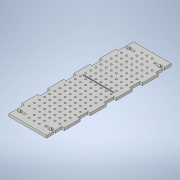
# Autodesk Inventor part: V3 Mounting Plate
Saved by Autodesk Inventor 2022.1 (Build 261234020, 234B)
## iProperties
Created: 2020-05-07
Part Number: V3 Mounting Plate
Material: Generic
Document SubType Name: Modeling
Designer: Workshop Tech
Density: 1 g/cm^3
Appearance: Default
Author: Workshop Tech
Autodesk Inventor part; units mm, degrees
ref_plane "YZ Plane" through (0, 0, 0) normal (1, 0, 0) x (0, 1, 0)
ref_plane "XZ Plane" through (0, 0, 0) normal (0, 1, 0) x (-1, 0, 0)
ref_plane "XY Plane" through (0, 0, 0) normal (0, 0, 1) x (1, 0, 0)
sketch "Sketch1" plane through (0, 0, 0) normal (0, 1, 0) x (-1, 0, 0)
  line L0 (0, 0) -> (104.96, 0)
  line L1 (104.96, 0) -> (104.96, -308.6568)
  line L2 (104.96, -308.6568) -> (0, -308.6568)
  line L3 (0, -308.6568) -> (0, 0)
  dimension "d0" = 104.96
  dimension "d1" = 308.6568
  constraints: 8 end point, 2 parallel, 1 horizontal, 1 perpendicular
  measures "d0" distance between parallel lines of L3 L1
  measures "d1" distance between parallel lines of L2 L0
extrude "Base" add sketch "Sketch1" along normal blind 6
sketch "Sketch7" plane through (0, 6, 0) normal (0, 1, 0) x (1, 0, 0)
  line L0 (0, 0) -> (0, 308.6568) projected
  line L1 (-104.96, 0) -> (0, 0) projected
  line L2 (-104.96, 0) -> (0, 0) projected
  line L3 (0, 0) -> (0, 308.6568) projected
  line L4 (0, 308.6568) -> (-104.96, 308.6568) projected
  line L5 (-104.96, 308.6568) -> (-104.96, 0) projected
  point P0 (-52.48, 270.5568)
  dimension "d35" = 38.1
  dimension "d36" = 52.48
  measures "d35" distance from line of L4 point (-52.48, 270.557)
  measures "d36" distance from line of L5 point (-52.48, 270.557)
hole "Board Hole" at (-52.48, 6, -270.5568) direction (0, -1, 0) diameter 4.25 end through all clearance for "Flat Head Machine Screw" size "M4" standard "Ansi Metric M Profile"
pattern_linear "Patterned Board Holes" count 19 spacing 12.7 along (0, 0, 1) count 7 spacing 12.7 along (1, 0, 0) of "Board Hole" second direction both ways yes
sketch "Sketch12" plane through (0, 6, 0) normal (0, 1, 0) x (1, 0, 0)
  line L0 (0, 308.6568) -> (0, 0) projected
  line L1 (-104.96, 0) -> (-104.96, 308.6568) projected
  line L2 (0, 0) -> (-5.875, 0)
  line L3 (-5.875, 0) -> (-5.875, 38.04)
  line L4 (-5.875, 38.04) -> (0, 38.04)
  line L5 (0, 38.04) -> (0, 0)
  line L6 (-104.96, 0) -> (0, 0) projected
  line L7 (-104.96, 0) -> (-99.085, 0)
  line L8 (-99.085, 0) -> (-99.085, 38.04)
  line L9 (-99.085, 38.04) -> (-104.96, 38.04)
  line L10 (-104.96, 38.04) -> (-104.96, 0)
  point P0 (0, 38.04)
  dimension "d188" = 5.875
  dimension "d189" = 38.04
  dimension "d190" = 5.875
  dimension "d191" = 38.04
  constraints: 16 end point, 4 parallel, 2 horizontal, 2 perpendicular
  measures "d188" distance of L3.end L4.end
  measures "d189" distance of L2.end L3.end
  measures "d190" distance of L9.end L8.end
  measures "d191" distance of L8.end L7.end
extrude "Extrusion4" cut sketch "Sketch12" against normal blind 25.4
sketch "Sketch13" plane through (0, 6, 0) normal (0, 1, 0) x (1, 0, 0)
  line L0 (0, 0) -> (0, 308.6568) projected
  line L1 (0, 308.6568) -> (-5.875, 308.6568)
  line L2 (-5.875, 270.6168) -> (0, 270.6168)
  line L3 (-5.875, 270.6168) -> (-5.875, 308.6568)
  line L4 (0, 308.6568) -> (0, 0) projected
  line L5 (0, 270.6168) -> (0, 308.6568)
  line L6 (0, 308.6568) -> (-104.96, 308.6568) projected
  line L7 (-104.96, 308.6568) -> (-99.085, 308.6568)
  line L8 (-99.085, 308.6568) -> (-99.085, 270.6168)
  line L9 (-99.085, 270.6168) -> (-104.96, 270.6168)
  line L10 (-104.96, 270.6168) -> (-104.96, 308.6568)
  point P0 (0, 38.1)
  point P1 (0, 270.6168)
  dimension "d175" = 38.04
  dimension "d176" = 5.875
  dimension "d178" = 5.875
  dimension "d179" = 38.04
  constraints: 16 end point, 2 horizontal, 2 parallel, 1 collinear, 1 perpendicular, 1 vertical
  measures "d175" distance of L2.start L1.end
  measures "d176" distance of L2.start L2.end
  measures "d178" distance of L8.end L9.end
  measures "d179" distance of L7.end L8.end
sketch "Sketch16" plane through (0, 6, 0) normal (0, 1, 0) x (1, 0, 0)
  circle A0 centre (-52.48, 270.5568) radius 2.125 projected
  point P0 (0, 0)
  point P1 (-52.48, 283.2568)
  dimension "d163" = 12.7
  measures "d163" distance of A0.centre point (-52.48, 283.257)
hole "Hole9" at (-52.48, 6, -283.2568) direction (0, -1, 0) diameter 4.25 end through all clearance for "Flat Head Machine Screw" size "M4" standard "Ansi Metric M Profile"
sketch "Sketch17" plane through (0, 6, 0) normal (0, 1, 0) x (1, 0, 0)
  line L0 (0, 38.04) -> (0, 308.6568) projected
  line L1 (-99.085, 0) -> (-5.875, 0) projected
  line L2 (0, 308.6568) -> (-104.96, 308.6568) projected
  line L3 (-5.875, 141.8134) -> (0, 141.8134)
  line L4 (0, 141.8134) -> (0, 166.8434)
  line L5 (0, 166.8434) -> (-5.875, 166.8434)
  line L6 (-5.875, 166.8434) -> (-5.875, 141.8134)
  line L7 (-52.48, 0) -> (-52.48, 308.6568)
  line L8 (-5.875, 206.2151) -> (0, 206.2151)
  line L9 (0, 206.2151) -> (0, 231.2451)
  line L10 (0, 231.2451) -> (-5.875, 231.2451)
  line L11 (-5.875, 231.2451) -> (-5.875, 206.2151)
  line L12 (-5.875, 77.4117) -> (0, 77.4117)
  line L13 (0, 77.4117) -> (0, 102.4417)
  line L14 (0, 102.4417) -> (-5.875, 102.4417)
  line L15 (-5.875, 102.4417) -> (-5.875, 77.4117)
  line L16 (-99.085, 141.8134) -> (-104.96, 141.8134)
  line L17 (-104.96, 141.8134) -> (-104.96, 166.8434)
  line L18 (-104.96, 166.8434) -> (-99.085, 166.8434)
  line L19 (-99.085, 166.8434) -> (-99.085, 141.8134)
  line L20 (-104.96, 231.2451) -> (-99.085, 231.2451)
  line L21 (-99.085, 231.2451) -> (-99.085, 206.2151)
  line L22 (-104.96, 206.2151) -> (-104.96, 231.2451)
  line L23 (-99.085, 206.2151) -> (-104.96, 206.2151)
  line L24 (-104.96, 102.4417) -> (-99.085, 102.4417)
  line L25 (-99.085, 102.4417) -> (-99.085, 77.4117)
  line L26 (-104.96, 77.4117) -> (-104.96, 102.4417)
  line L27 (-99.085, 77.4117) -> (-104.96, 77.4117)
  point P0 (-52.48, 154.3284)
  point P1 (-5.875, 154.3284)
  point P2 (-52.48, 154.3284)
  point P3 (0, 154.3284)
  point P4 (-5.875, 218.7301)
  point P5 (0, 218.7301)
  point P6 (-5.875, 89.9267)
  point P7 (0, 89.9267)
  point P8 (-104.96, 102.6267)
  point P9 (-104.96, 231.4301)
  point P10 (-99.085, 154.3284)
  point P11 (-104.96, 154.3284)
  point P12 (-99.085, 218.7301)
  point P13 (-104.96, 218.7301)
  point P14 (-99.085, 89.9267)
  point P15 (-104.96, 89.9267)
  dimension "d257" = 5.875
  dimension "d258" = 25.03
  dimension "d259" = 5.875
  dimension "d260" = 25.03
  dimension "d261" = 5.875
  dimension "d262" = 25.03
  dimension "d264" = 89.9267
  dimension "d266" = 89.9267
  dimension "d269" = 154.3284
  dimension "d270" = 52.48
  constraints: 50 end point, 18 symmetric about line, 9 midpoint, 6 parallel, 3 horizontal, 3 perpendicular, 3 point on line, 1 horizontal alignment
  measures "d257" distance of L5.end L4.end
  measures "d258" distance of L4.end L3.end
  measures "d259" distance of L10.end L10.start
  measures "d260" distance of L10.start L9.start
  measures "d261" distance of L14.end L14.start
  measures "d262" distance of L14.start L13.start
  measures "d264" distance from line of L2 point (0, 218.73)
  measures "d266" distance from line of L1 point (-5.875, 89.927)
  measures "d269" distance from line of point (-52.48, 154.328) L2
  measures "d270" distance from line of point (-52.48, 154.328) L0
extrude "Extrusion6" cut sketch "Sketch17" against normal blind 25.4
extrude "Extrusion7" cut sketch "Sketch13" against normal blind 25.4
sketch "Sketch18" plane through (0, 6, 0) normal (0, 1, 0) x (1, 0, 0)
  line L0 (0, 291.6047) -> (0, 287.1089) projected
  line L1 (0, 291.6047) -> (0, 287.1089) projected
  line L2 (-28.125, 287.2339) -> (-28.125, 291.7297)
  line L3 (0, 291.7297) -> (0, 287.1089)
  line L4 (-16.25, 285.2943) -> (-12, 285.2943)
  line L5 (-12, 293.5443) -> (-16.25, 293.5443)
  line L6 (0, 287.1089) -> (-12, 287.1089)
  line L7 (-16.25, 287.2339) -> (-28.125, 287.2339)
  line L8 (-28.125, 291.7297) -> (-16.25, 291.7297)
  line L9 (-12, 291.7297) -> (0, 291.7297)
  line L10 (-16.25, 293.5443) -> (-16.25, 291.7297)
  line L11 (-16.25, 287.2339) -> (-16.25, 285.2943)
  line L12 (-12, 285.2943) -> (-12, 287.1089)
  line L13 (-12, 291.7297) -> (-12, 293.5443)
  line L14 (-5.875, 308.6568) -> (-99.085, 308.6568) projected
  line L15 (-99.085, 38.04) -> (-99.085, 0) projected
  line L16 (-99.085, 308.6568) -> (-99.085, 270.6168) projected
  line L17 (-52.48, 308.6568) -> (-52.48, 0)
  line L18 (-142.1882, 0) -> (-142.1882, 308.6568)
  line L19 (-142.1882, 154.3284) -> (31.2958, 154.3284)
  line L20 (-104.96, 291.6047) -> (-104.96, 287.1089)
  line L21 (-104.96, 291.6047) -> (-104.96, 287.1089)
  line L22 (-76.835, 287.2339) -> (-76.835, 291.7297)
  line L23 (-104.96, 291.7297) -> (-104.96, 287.1089)
  line L24 (-88.71, 285.2943) -> (-92.96, 285.2943)
  line L25 (-92.96, 293.5443) -> (-88.71, 293.5443)
  line L26 (-104.96, 287.1089) -> (-92.96, 287.1089)
  line L27 (-88.71, 287.2339) -> (-76.835, 287.2339)
  line L28 (-76.835, 291.7297) -> (-88.71, 291.7297)
  line L29 (-92.96, 291.7297) -> (-104.96, 291.7297)
  line L30 (-88.71, 293.5443) -> (-88.71, 291.7297)
  line L31 (-88.71, 287.2339) -> (-88.71, 285.2943)
  line L32 (-92.96, 285.2943) -> (-92.96, 287.1089)
  line L33 (-92.96, 291.7297) -> (-92.96, 293.5443)
  line L34 (-99.085, 308.6568) -> (-5.875, 308.6568)
  line L35 (0, 17.0521) -> (0, 21.5479)
  line L36 (0, 17.0521) -> (0, 21.5479)
  line L37 (-28.125, 21.4229) -> (-28.125, 16.9271)
  line L38 (0, 16.9271) -> (0, 21.5479)
  line L39 (-16.25, 23.3625) -> (-12, 23.3625)
  line L40 (-12, 15.1125) -> (-16.25, 15.1125)
  line L41 (0, 21.5479) -> (-12, 21.5479)
  line L42 (-16.25, 21.4229) -> (-28.125, 21.4229)
  line L43 (-28.125, 16.9271) -> (-16.25, 16.9271)
  line L44 (-12, 16.9271) -> (0, 16.9271)
  line L45 (-16.25, 15.1125) -> (-16.25, 16.9271)
  line L46 (-16.25, 21.4229) -> (-16.25, 23.3625)
  line L47 (-12, 23.3625) -> (-12, 21.5479)
  line L48 (-12, 16.9271) -> (-12, 15.1125)
  line L49 (-99.085, 0) -> (-99.085, 38.04)
  line L50 (-76.835, 16.9271) -> (-88.71, 16.9271)
  line L51 (-76.835, 21.4229) -> (-76.835, 16.9271)
  line L52 (-88.71, 21.4229) -> (-76.835, 21.4229)
  line L53 (-92.96, 15.1125) -> (-88.71, 15.1125)
  line L54 (-92.96, 16.9271) -> (-92.96, 15.1125)
  line L55 (-88.71, 21.4229) -> (-88.71, 23.3625)
  line L56 (-92.96, 23.3625) -> (-92.96, 21.5479)
  line L57 (-88.71, 23.3625) -> (-92.96, 23.3625)
  line L58 (-92.96, 16.9271) -> (-104.96, 16.9271)
  line L59 (-104.96, 21.5479) -> (-92.96, 21.5479)
  line L60 (-104.96, 17.0521) -> (-104.96, 21.5479)
  line L61 (-104.96, 17.0521) -> (-104.96, 21.5479)
  line L62 (-104.96, 16.9271) -> (-104.96, 21.5479)
  line L63 (-88.71, 15.1125) -> (-88.71, 16.9271)
  point P0 (-5.875, 270.6168)
  point P1 (-19.9732, 289.3568)
  point P2 (0, 289.3568)
  point P3 (0, 289.3568)
  point P4 (-84.9868, 289.3568)
  point P5 (-104.96, 289.3568)
  point P6 (-104.96, 289.3568)
  point P7 (-5.875, 38.04)
  point P8 (-19.9732, 19.3)
  point P9 (0, 19.3)
  point P10 (0, 19.3)
  point P11 (-84.9868, 19.3)
  point P12 (-104.96, 19.3)
  point P13 (-104.96, 19.3)
  dimension "d237" = 28.125
  dimension "d238" = 4.25
  dimension "d239" = 8.25
  dimension "d240" = 12
  dimension "d242" = 16.9271
  dimension "d256" = 4.4958
  constraints: 118 end point, 52 symmetric about line, 10 parallel, 8 midpoint, 4 horizontal, 4 perpendicular, 2 equal length, 1 horizontal alignment, 1 vertical
  measures "d237" distance of L2.end L3.start
  measures "d238" distance of L5.end L5.start
  measures "d239" distance of L5.start L4.end
  measures "d240" distance of L9.start L3.start
  measures "d242" distance between parallel lines of L14 L9
  measures "d256" distance between parallel lines of L8 L7
extrude "Extrusion8" cut sketch "Sketch18" against normal blind 25.4
pattern_linear "Rectangular Pattern6" count 2 spacing 12.7 along (0, 0, -1) count 3 spacing 12.7 along (-1, 0, 0) of "Hole9" second direction both ways yes
sketch "Sketch19" plane through (0, 6, 0) normal (0, 1, 0) x (1, 0, 0)
  circle A0 centre (-52.48, 29.0068) radius 1.6256
  circle A1 centre (-52.48, 41.9568) radius 2.125 projected
  point P0 (0, 0)
  dimension "d225" = 3.2512
  constraints: 1 centre point, 1 vertical alignment
  measures "d225" diameter of A0
sketch "Sketch20" plane through (0, 6, 0) normal (0, 1, 0) x (1, 0, 0)
  line L0 (-14.38, 176.5768) -> (-90.58, 176.5768)
  line L1 (-90.58, 176.5768) -> (-90.58, 174.0368)
  line L2 (-90.58, 174.0368) -> (-14.38, 174.0368)
  line L3 (-14.38, 174.0368) -> (-14.38, 176.5768)
  line L4 (-5.875, 77.4117) -> (-5.875, 102.4417) projected
  circle A0 centre (-52.48, 168.9568) radius 2.125 projected
  point P0 (0, 0)
  dimension "d234" = 2.54
  dimension "d271" = 76.2
  dimension "d272" = 8.505
  dimension "d273" = 5.08
  constraints: 8 end point, 2 parallel, 1 horizontal, 1 perpendicular
  measures "d234" distance of L1.end L0.end
  measures "d271" distance of L0.start L0.end
  measures "d272" distance between parallel lines of L4 L3
  measures "d273" distance from line of L2 A0.centre
extrude "Extrusion10" cut sketch "Sketch20" against normal blind 1 contours L3 L2 L1 L0
hole "Hole10" at (-52.48, 6, -29.0068) direction (0, -1, 0) diameter 4.25 end through all clearance for "Flat Head Machine Screw" size "M4" standard "Ansi Metric M Profile"
pattern_linear "Rectangular Pattern8" count 3 spacing 12.7 along (1, 0, 0) count 2 spacing 12.7 along (0, 0, 1) of "Hole10" first direction both ways yes
equation "\"d191\" = d189"
body "Solid1"
